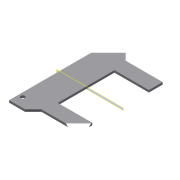
# Autodesk Inventor part: bottom_sensor
Saved by Autodesk Inventor 2014 (Build 180170000, 170)
## iProperties
Created: 2014-01-08
Part Number: bottom_sensor
Material: Generisch
Document SubType Name: Modeling
Designer: Felix
Density: 1 g/cm^3
Appearance: Vorgabe
Author: Felix
Autodesk Inventor part; units mm, degrees
note: some values were not read from the file. Chosen so that the rebuilt part matches the saved one: sketch regions of "Extrusion1".
ref_plane "YZ Plane" through (0, 0, 0) normal (1, 0, 0) x (0, 1, 0)
ref_plane "XZ Plane" through (0, 0, 0) normal (0, 1, 0) x (-1, 0, 0)
ref_plane "XY Plane" through (0, 0, 0) normal (0, 0, 1) x (1, 0, 0)
sketch "Skizze1" plane through (0, 0, 0) normal (0, 0, 1) x (1, 0, 0)
  arc A0 (3, 7) -> (-3, 1) centre (3, 1) ccw projected
  line L0 (16.5, 7) -> (3, 7) projected
  line L1 (16.5, 7) -> (40.4545, 7) projected
  line L2 (-3, 0) -> (-3, -59.5) projected
  line L3 (-3, 1) -> (-3, 0) projected
  arc A1 (-3, -60.5) -> (3, -66.5) centre (3, -60.5) ccw projected
  line L4 (-3, -59.5) -> (-3, -60.5) projected
  line L5 (3, -66.5) -> (16.5, -66.5) projected
  line L6 (16.5, -56.3086) -> (5, -56.3086) projected
  line L7 (27, -49) -> (27, -62.5) projected
  line L8 (27, -49) -> (16.5, -49) projected
  line L9 (16.5, -49) -> (16.5, -56.3086) projected
  line L10 (16.5, -56.3086) -> (5, -56.3086) projected
  line L11 (5, -56.3086) -> (5, -37.5) projected
  line L12 (5, -37.5) -> (3, -37.5) projected
  line L13 (3, -37.5) -> (3, -22) projected
  line L14 (3, -22) -> (5, -22) projected
  line L15 (5, -22) -> (5, -3.0505) projected
  line L16 (5, -3.0505) -> (16.5, -3.0505) projected
  line L17 (16.5, -3.0505) -> (16.5, -10.5) projected
  line L18 (27, -10.5) -> (16.5, -10.5) projected
  line L19 (27, 3) -> (27, -10.5) projected
  line L20 (27, 3) -> (16.5, 3) projected
  line L21 (16.5, 3) -> (16.5, 7) projected
  line L22 (16.5, 7) -> (3, 7) projected
  arc A2 (3, 7) -> (-3, 1) centre (3, 1) ccw projected
  line L23 (-3, 1) -> (-3, 0) projected
  circle A3 centre (0, 0) radius 3 projected
  line L24 (-3, 0) -> (-3, -59.5) projected
  circle A4 centre (0, -59.5) radius 3 projected
  line L25 (-3, -59.5) -> (-3, -60.5) projected
  arc A5 (-3, -60.5) -> (3, -66.5) centre (3, -60.5) ccw projected
  line L26 (3, -66.5) -> (16.5, -66.5) projected
  line L27 (16.5, -66.5) -> (16.5, -62.5) projected
  line L28 (16.5, -62.5) -> (27, -62.5) projected
  line L29 (-3, 7) -> (16.5, 7)
  line L30 (16.5, -66.5) -> (-3, -66.5)
  line L31 (-3, -66.5) -> (-3, 7)
  line L32 (16.5, 7) -> (41.6272, 7)
  line L33 (41.6272, 7) -> (41.6272, -9.0628)
  line L34 (41.6272, -9.0628) -> (16.5, -9.0628)
  line L35 (16.5, -66.5) -> (41.6272, -66.5)
  line L36 (41.6272, -66.5) -> (41.6272, -50.4372)
  line L37 (41.6272, -50.4372) -> (16.5, -50.4372)
  circle A6 centre (0, 0) radius 1.5 projected
  circle A7 centre (0, -59.5) radius 1.5 projected
  line L38 (16.5, -50.4372) -> (16.5, -9.0628)
  point P0 (0, 0)
  dimension "d5" = 7
  dimension "d6" = 7
  constraints: 20 end point, 3 horizontal, 3 parallel, 2 collinear, 2 perpendicular, 1 point on line
  measures "d5" distance from line of L29 A3.centre
  measures "d6" distance from line of L30 A7.centre
extrude "Extrusion1" add sketch "Skizze1" along normal blind 1.6 contours A3 | A4 | L0 L21 L20 L19 L34 L17 L16 L15 L14 L13 L12 L11 L6 L9 L37 L7 L28 L27 L5 A1 L4 L2 L3 A0 | A0 L31 L29 | L1 L32 L33 L34 L19 L20 L21 | A1 L30 L31 | L17 L38 L9 L6 L11 L12 L13 L14 L15 L16 | L27 L28 L7 L37 L36 L35
sketch "Skizze2" plane through (0, 0, 1.6) normal (0, 0, 1) x (1, 0, 0)
  line L0 (-3, -66.5) -> (41.6272, -66.5) projected
  line L1 (41.6272, -9.0628) -> (41.6272, 7) projected
  line L2 (41.6272, 7) -> (-3, 7) projected
  line L3 (41.6272, 2) -> (14.5797, 2)
  line L4 (14.5797, 2) -> (9.5797, 7)
  line L5 (14.5797, 2) -> (21.6508, 2) construction
  dimension "d2" = 135
  dimension "d7" = 5
  constraints: 6 end point, 2 parallel, 2 point on line, 1 equal length, 1 horizontal
  measures "d2" angle of L5 L4
  measures "d7" distance between parallel lines of L2 L3
extrude "Extrusion2" cut sketch "Skizze2" against normal through all
ref_plane "Arbeitsebene1" through (-3, -29.75, 1.6) normal (0, 1, 0) x (1, 0, 0)
mirror "Spiegeln1" about plane through (-3, -29.75, 1.6) normal (0, 1, 0) of "Extrusion2"
